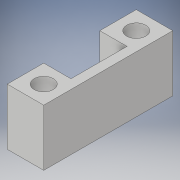
# Autodesk Inventor part: 3710-lasers
Saved by Autodesk Inventor 2019 (Build 230136000, 136)
## iProperties
Created: 2022-12-05
Part Number: 3710-lasers
Material: Generic
Document SubType Name: Modeling
Designer: Ella Moss
Density: 1 g/cm^3
Appearance: Default
Author: Ella Moss
Autodesk Inventor part; units mm, degrees
ref_plane "YZ Plane" through (0, 0, 0) normal (1, 0, 0) x (0, 1, 0)
ref_plane "XZ Plane" through (0, 0, 0) normal (0, 1, 0) x (-1, 0, 0)
ref_plane "XY Plane" through (0, 0, 0) normal (0, 0, 1) x (1, 0, 0)
sketch "Sketch1" plane through (0, 0, 0) normal (0, 1, 0) x (-1, 0, 0)
  line L0 (20.0152, 35.4076) -> (0, 35.4076)
  line L1 (0, 35.4076) -> (0, -35.4076)
  line L2 (0, -35.4076) -> (20.0152, -35.4076)
  circle A0 centre (10.0076, 25.4) radius 5.25
  circle A1 centre (10.0076, -25.4) radius 5.25
  line L3 (20.0152, 15.3924) -> (5.08, 15.3924)
  line L4 (5.08, 15.3924) -> (5.08, -15.3924)
  line L5 (5.08, -15.3924) -> (20.0152, -15.3924)
  line L6 (20.0152, -35.4076) -> (20.0152, -15.3924)
  line L7 (20.0152, 15.3924) -> (20.0152, 35.4076)
  point P0 (0, 0)
  point P1 (0, 0)
  dimension "d1" = 10.5
  dimension "d2" = 10.5
  dimension "d3" = 50.8
  dimension "d4" = 10.0076
  dimension "d5" = 10.0076
  dimension "d6" = 10.0076
  dimension "d7" = 5.08
  dimension "d9" = 10.0076
  dimension "d10" = 10.0076
  dimension "d11" = 10.0076
  constraints: 16 end point, 4 perpendicular, 3 parallel, 2 centre point, 2 coincident, 2 horizontal, 2 vertical alignment, 1 midpoint
  measures "d1" diameter of A1
  measures "d2" diameter of A0
  measures "d3" distance of A1.centre A0.centre
  measures "d4" distance from line of L0 A0.centre
  measures "d5" distance from line of L2 A1.centre
  measures "d6" distance from line of L1 A1.centre
  measures "d7" distance between parallel lines of L1 L4
  measures "d9" distance from line of A0.centre L3
  measures "d10" distance from line of A1.centre L5
  measures "d11" distance from line of L7 A0.centre
extrude "Extrusion1" add sketch "Sketch1" along normal blind 31
body "Solid1"
